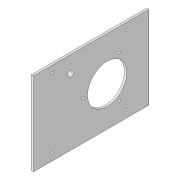
# Autodesk Inventor part: BREEZE-M08
Saved by Autodesk Inventor 2020 (Build 240168000, 168)
## iProperties
Created: 2020-04-12
Part Number: BREEZE-M08
Material: Generic
Description: AIR INLET PANEL
Document SubType Name: Modeling
Designer: John K
Density: 1 g/cm^3
Appearance: Default
Author: John K
Autodesk Inventor part; units mm, degrees
ref_plane "YZ Plane" through (0, 0, 0) normal (1, 0, 0) x (0, 1, 0)
ref_plane "XZ Plane" through (0, 0, 0) normal (0, 1, 0) x (-1, 0, 0)
ref_plane "XY Plane" through (0, 0, 0) normal (0, 0, 1) x (1, 0, 0)
sketch "Face" plane through (0, 0, 0) normal (0, 0, 1) x (1, 0, 0)
  circle A0 centre (143.9602, -80.6846) radius 6.35
  circle A1 centre (39.7975, -186.0352) radius 2.4
  circle A2 centre (85.2205, -107.3602) radius 2.4
  circle A3 centre (130.6435, -186.0352) radius 2.4
  circle A4 centre (85.2205, -159.8102) radius 42.45
  circle A5 centre (14.75, -202.58) radius 2.6
  circle A6 centre (165.25, -202.58) radius 2.6
  circle A7 centre (14.75, -40.38) radius 2.6
  circle A8 centre (165.25, -40.38) radius 2.6
  line L0 (180, 0) -> (0, 0)
  line L1 (0, 0) -> (0, -250)
  line L2 (0, -250) -> (180, -250)
  line L3 (180, -250) -> (180, 0)
  point P0 (94.9979, -134.0949)
  point P1 (175.25, -245.25)
sketch "Sketch1" plane through (0, 0, 0) normal (1, 0, 0) x (0, 1, 0)
  circle A0 centre (53.9602, 44.3154) radius 6.35
  circle A1 centre (-50.2025, -61.0352) radius 2.4
  circle A2 centre (-4.7795, 17.6398) radius 2.4
  circle A3 centre (40.6435, -61.0352) radius 2.4
  circle A4 centre (-4.7795, -34.8102) radius 42.45
  circle A5 centre (-75.25, -77.58) radius 2.6
  circle A6 centre (75.25, -77.58) radius 2.6
  circle A7 centre (-75.25, 84.62) radius 2.6
  circle A8 centre (75.25, 84.62) radius 2.6
  line L0 (90, 125) -> (-90, 125)
  line L1 (-90, 125) -> (-90, -125)
  line L2 (-90, -125) -> (90, -125)
  line L3 (90, -125) -> (90, 125)
  point P0 (0, 0)
  point P1 (-90, 0)
  point P2 (0, 125)
  constraints: 1 horizontal alignment, 1 vertical alignment, 2 other
extrude "Extrusion1" add sketch "Sketch1" along normal mid plane 4.75
sketch "Sketch2" plane through (2.375, 0, 0) normal (1, 0, 0) x (0, 0, -1)
  circle A0 centre (-17.6398, -4.7795) radius 2.4 projected
  circle A1 centre (61.0352, -50.2025) radius 2.4 projected
  circle A2 centre (61.0352, 40.6435) radius 2.4 projected
  point P0 (0, 0)
hole "Hole1" at (2.375, -4.7795, 17.6398) at (2.375, -50.2025, -61.0352) at (2.375, 40.6435, -61.0352) direction (-1, 0, 0) diameter 5.5 end through all clearance for "Socket Head Cap Screw" size "M5" standard "Ansi Metric M Profile"
body "Solid1"
